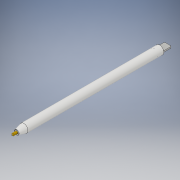
# Autodesk Inventor part: Pencil Body
Saved by Autodesk Inventor 2018 (Build 220112000, 112)
## iProperties
Created: 2020-01-09
Part Number: Pencil Body
Material: Generic
Document SubType Name: Modeling
Designer: AOFUser
Density: 1 g/cm^3
Appearance: Smooth - White
Author: AOFUser
Autodesk Inventor part; units mm, degrees
ref_plane "YZ Plane" through (0, 0, 0) normal (1, 0, 0) x (0, 1, 0)
ref_plane "XZ Plane" through (0, 0, 0) normal (0, 1, 0) x (-1, 0, 0)
ref_plane "XY Plane" through (0, 0, 0) normal (0, 0, 1) x (1, 0, 0)
sketch "Sketch1" plane through (0, 0, 0) normal (0, 1, 0) x (-1, 0, 0)
  line L0 (0, 0) -> (0, -152.4)
  line L1 (0, 0) -> (0, 5.08)
  line L2 (0, 5.08) -> (1.27, 5.08)
  line L3 (1.27, 5.08) -> (1.27, 0)
  line L4 (1.27, 0) -> (0, 0)
  line L5 (0, 0) -> (0, -4.826)
  line L6 (0, -4.826) -> (1.397, -4.826)
  line L7 (1.397, -4.826) -> (1.397, 0)
  line L8 (1.397, 0) -> (1.27, 0)
  line L9 (0, 0) -> (0, -7.62)
  line L10 (4.445, -7.62) -> (2.54, 0)
  line L11 (4.445, -152.4) -> (4.445, -7.62)
  line L12 (2.54, 0) -> (2.2936, -0.0616)
  line L13 (2.2936, -0.0616) -> (4.1986, -7.6816)
  line L14 (4.1986, -7.6816) -> (4.1986, -152.4)
  line L15 (4.1986, -152.4) -> (4.445, -152.4)
  line L16 (1.397, -4.826) -> (4.1986, -7.6816)
  line L17 (0, -152.4) -> (3.81, -152.4)
  line L18 (3.81, -152.4) -> (3.81, -146.304)
  line L19 (3.81, -146.304) -> (0, -146.304)
  line L20 (3.81, -146.304) -> (4.445, -146.304)
  dimension "d0" = 152.4
  dimension "d1" = 5.08
  dimension "d2" = 1.27
  dimension "d3" = 4.826
  dimension "d4" = 1.397
  dimension "d5" = 2.54
  dimension "d6" = 7.62
  dimension "d7" = 4.445
  dimension "d8" = 4.445
  dimension "d9" = 0.254
  dimension "d10" = 3.81
  dimension "d11" = 6.096
  dimension "d21" = 0.2464
  constraints: 42 end point, 5 perpendicular, 5 point on line, 3 vertical, 2 horizontal, 1 collinear, 1 parallel
  measures "d0" distance of L0.start L0.end
  measures "d1" distance of L0.start L1.end
  measures "d2" distance of L1.end L2.end
  measures "d3" distance of L0.start L5.end
  measures "d4" distance of L5.end L6.end
  measures "d5" distance of L0.start L10.end
  measures "d6" distance of L0.start L9.end
  measures "d7" distance of L9.end L10.start
  measures "d8" distance of L0.end L11.start
  measures "d9" distance of L10.end L12.end
  measures "d10" distance of L0.end L17.end
  measures "d11" distance of L17.end L18.end
  measures "d21" distance between parallel lines of L11 L14
revolve "Revolution1" add sketch "Sketch1" angle 360 about axis through (0, 0, 0) along (0, 0, -1)
sketch "Sketch2" plane through (0, 0, -152.4) normal (0, 0, -1) x (-1, 0, 0)
  line L0 (0, 0) -> (0, -0.762)
  line L1 (0, -0.762) -> (3.733, -0.762)
  circle A0 centre (0, 0) radius 3.81 projected
  line L2 (0, -0.762) -> (-3.733, -0.762)
  line L3 (0, 0) -> (0, 0.762)
  line L4 (0, 0.762) -> (3.733, 0.762)
  line L5 (0, 0.762) -> (-3.733, 0.762)
  dimension "d13" = 0.762
  dimension "d14" = 0.762
  constraints: 12 end point, 4 point on circle, 2 perpendicular, 2 vertical, 1 horizontal, 1 point on line
  measures "d13" distance of L0.start L0.end
  measures "d14" distance of L3.start L3.end
extrude "Extrusion1" add sketch "Sketch2" along normal blind 8.89 contours L3 L4 A0 L1 L0 | L0 L2 A0 L5 L3
fillet "Fillet1" radius 1.016 4 edges at (-3.81, 0, -161.29) (3.81, 0, -161.29) (0, 0.762, -152.4) (0, -0.762, -152.4)
chamfer "Chamfer1" distance 1.016 distance2 0.508 1 edges at (1.27, 0, 5.08) measured on face at (-1.2659, -0.1022, 1.6933)
sketch "Sketch3" plane through (-3.733, -0.762, -153.416) normal (0, -1, 0) x (1, 0, 0)
  point P0 (3.733, 153.416)
body "Solid1"
